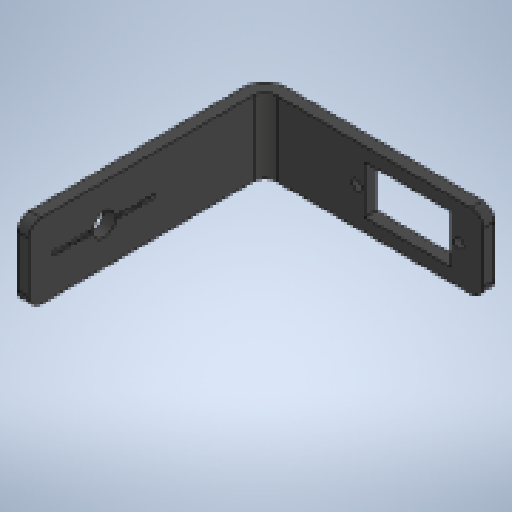
# Autodesk Inventor part: Topplate
Saved by Autodesk Inventor 2023.4 (Build 274418000, 418)
## iProperties
Created: 2024-05-24
Part Number: Topplate
Material: Generic
Document SubType Name: Modeling
Designer: Nathan Cai
Mass: 5.74421 g
Surface Area: 49.0442 cm^2
Volume: 5.74421 cm^3
Density: 1 g/cm^3
Appearance: Rubber - Black
Author: Nathan Cai
Autodesk Inventor part; units mm, degrees
ref_plane "YZ Plane" through (0, 0, 0) normal (1, 0, 0) x (0, 1, 0)
ref_plane "XZ Plane" through (0, 0, 0) normal (0, 1, 0) x (-1, 0, 0)
ref_plane "XY Plane" through (0, 0, 0) normal (0, 0, 1) x (1, 0, 0)
sketch "Sketch1" plane through (0, 0, 0) normal (1, 0, 0) x (0, 1, 0)
  circle A0 centre (0, 0) radius 2.5 construction
  circle A1 centre (0, 0) radius 3
  line L0 (0, 0) -> (0, -32.9) construction
  line L1 (-10, -85.8) -> (10, -85.8)
  line L2 (10, -85.8) -> (10, 20)
  line L3 (10, 20) -> (-10, 20)
  line L4 (-10, 20) -> (-10, -85.8)
  line L5 (-10, -85.8) -> (10, 20) construction
  line L6 (10, -85.8) -> (-10, 20) construction
  circle A2 centre (0, 0) radius 4.25 construction
  circle A3 centre (0, -4.25) radius 0.625
  circle A4 centre (0, -6) radius 0.625
  circle A5 centre (0, -7.75) radius 0.625
  circle A6 centre (0, -9.5) radius 0.625
  circle A7 centre (0, -11.25) radius 0.625
  circle A8 centre (0, -13) radius 0.625
  circle A9 centre (0, 13) radius 0.625
  circle A10 centre (0, 11.25) radius 0.625
  circle A11 centre (0, 9.5) radius 0.625
  circle A12 centre (0, 7.75) radius 0.625
  circle A13 centre (0, 6) radius 0.625
  circle A14 centre (0, 4.25) radius 0.625
  line L7 (-6.4, -54.3) -> (6.4, -54.3)
  line L8 (6.4, -54.3) -> (6.4, -77.3)
  line L9 (6.4, -77.3) -> (-6.4, -77.3)
  line L10 (-6.4, -77.3) -> (-6.4, -54.3)
  line L11 (-6.4, -54.3) -> (6.4, -77.3) construction
  line L12 (6.4, -54.3) -> (-6.4, -77.3) construction
  circle A15 centre (0, -65.8) radius 13.65 construction
  circle A16 centre (0, -79.45) radius 1.3
  circle A17 centre (0, -52.15) radius 1.3
  dimension "d5" = 8.5
  dimension "d19" = 27.3
  dimension "d0" = 5
  dimension "d1" = 6
  dimension "d2" = 20
  dimension "d3" = 105.8
  dimension "d4" = 20
  dimension "d6" = 1.25
  dimension "d9" = 1.75
  dimension "d16" = 360
  dimension "d18" = 23
  dimension "d20" = 2.6
  dimension "d21" = 12.8
  dimension "d24" = 360
  dimension "d26" = 20
  constraints: 26 end point, 16 centre point, 4 coincident, 4 midpoint, 4 parallel, 3 point on line, 2 horizontal, 2 perpendicular, 2 vertical, 2 vertical alignment, 44 other
  measures "d0" diameter of A0
  measures "d1" diameter of A1
  measures "d2" distance of L3.end L2.end
  measures "d3" distance of L2.end L1.end
  measures "d4" distance from line of L3 L0.start
  measures "d6" diameter of A3
  measures "d9" distance of A3.centre A4.centre
  measures "d18" distance between parallel lines of L7 L9
  measures "d20" diameter of A16
  measures "d21" distance between parallel lines of L10 L8
  measures "d26" distance from line of L1 point (0, -65.8)
extrude "Extrusion1" add sketch "Sketch1" along normal blind 3.175
fillet "Fillet1" radius 3.175 4 edges at (1.5875, 10, 20) (1.5875, -10, 20) (1.5875, 10, -85.8) (1.5875, -10, -85.8)
sketch "Sketch2" plane through (3.175, 0, 0) normal (1, 0, 0) x (0, 0, -1)
  line L0 (82.625, 10) -> (-16.825, 10) projected
  line L1 (40, 10) -> (40, -10)
  line L2 (-16.825, -10) -> (82.625, -10) projected
  line L3 (-20, 6.825) -> (-20, -6.825) projected
  point P0 (0, 0)
  dimension "d30" = 60
  constraints: 2 end point, 2 point on line, 1 vertical
  measures "d30" distance between parallel lines of L3 L1
bend part "Bend Part1" radius 3 angle 90 line through (3.175, 10, -40) along (0, -1, 0) centre toward (1, 0, 0) moving side (0, 0, -1) both sides no
body "Solid1"
